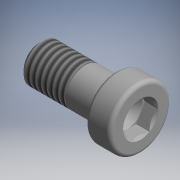
# Autodesk Inventor part: DIN-6912 - M10x20(F)
Saved by Autodesk Inventor 2017.3 (Build 213256000, 256)
## iProperties
Part Number: DIN-6912 - M10x20(F)
Material: Generic
Catalog Web Link: www.cadenas.de
Description: DIN-6912-Hexagon socket head cap screw with centre hole and low head
Vendor: FESTO
Document SubType Name: Modeling
Designer: partserver
Manufacturer: FESTO
Mass: 2.53132 g
Surface Area: 14.4572 cm^2
Volume: 2.53132 cm^3
Density: 1 g/cm^3
Appearance: PSOLRGB-192-192-192
Category: PARTsolutions
Company: FESTO
Title: DIN-6912 - M10x20(F)
Author: Cadenas PARTsolutions
Comments: Hexagon socket head cap screw with centre hole and low head
PSOL_IDENT_0: {$CADENAS_DATA\23d-libs\festo\zyl_zubeh\din_6912\din_6912.prj},183 {VTYP=3D},{NB=DIN-6912 - M10x20(F
PSOL_IDENT_1: )},{LINA=DIN-6912 - M10x20(F)},{NN=DIN-6912},{DATE=16.11.2017 11:29:57},{GEOMDATE=16.11.2017 11:29:4
PSOL_IDENT_2: 4},{VERSION=},{LINEID=430},{WBVAR=},{WBNUMERIC=}  {NB=DIN-6912 - M10x20(F)},{LINA=DIN-6912 - M10x20(
PSOL_IDENT_3: F)},{KT=L},{IDNR=},{NENN=M10x20},{D=10.000},{L=20.000},{DK=8.160},{LS=3.500},{LG=8.000},{DK1=16.000}
PSOL_IDENT_4: ,{DH=5.000},{K=6.500},{R=0.400},{V=1.000},{S=8.000},{T1=3.500},{T2=7.500},{F=1.020},{DA=11.200},{DW=
PSOL_IDENT_5: 15.030}
NB: DIN-6912 - M10x20(F)
NN: DIN-6912
NT: Hexagon socket head cap screw with centre hole and low head
NBSYN: DIN-6912 - $NENN.(F)
LINA: DIN-6912 - M10x20(F)
CATALOG: Festo
ROWDESC: M10x20
D: 10
L: 20
DK: 8.16
LS: 3.5
LG: 8
DK1: 16
DH: 5
K: 6.5
R: 0.4
V: 1
S: 8
T1: 3.5
T2: 7.5
F: 1.02
DA: 11.2
DW: 15.03
SUPPLIER: FESTO
ARTICLENO: DIN-6912 - M10x20(F)
BOMINFO: DIN-6912 - M10x20(F)
CREATOR: CADENAS GmbH
Autodesk Inventor part; units mm, degrees
sketch "Sketch_1" plane through (0, 0, 0) normal (0, 0, 1) x (1, 0, 0)
  line L0 (20, 0) -> (3.5, 0)
  line L1 (3.5, 0) -> (1, 2.5)
  line L2 (1, 2.5) -> (-1.5, 2.5)
  line L3 (-1.5, 2.5) -> (-3, 4)
  line L4 (-3, 4) -> (-5.8812, 4)
  line L5 (-5.8812, 4) -> (-6.5, 4.6188)
  line L6 (-6.5, 4.6188) -> (-6.5, 7)
  arc A0 (-5.5, 8) -> (-6.5, 7) centre (-5.5, 7) ccw
  line L7 (-5.5, 8) -> (-1, 8)
  arc A1 (0, 7) -> (-1, 8) centre (-1, 7) ccw
  line L8 (0, 7) -> (0, 5)
  line L9 (0, 5) -> (19.08, 5)
  line L10 (19.08, 5) -> (20, 4.08)
  line L11 (20, 4.08) -> (20, 0)
  line L12 (20, 0) -> (3.5, 0)
  constraints: 26 end point, 4 point on circle, 2 centre point
revolve "Revolution1" add sketch "Sketch_1" angle 360 about axis through (20, 0, 0) along (-1, 0, 0)
thread "Thread1" size "M10x1.5" class "6g" standard "ISO Metric profile" length 11.08
sketch "Sketch_2" plane through (-6.5, 0, 0) normal (1, 0, 0) x (0, 0, -1)
  line L0 (-4, -2.3094) -> (0, -4.6188)
  line L1 (0, -4.6188) -> (4, -2.3094)
  line L2 (4, -2.3094) -> (4, 2.3094)
  line L3 (4, 2.3094) -> (0, 4.6188)
  line L4 (0, 4.6188) -> (-4, 2.3094)
  line L5 (-4, 2.3094) -> (-4, -2.3094)
  constraints: 12 end point
extrude "Extrusion1" cut sketch "Sketch_2" along normal blind 3.5
ref_plane "MONTAGE_XY" through (0, 0, 0) normal (1, 0, 0) x (0, 0, -1)
ref_plane "MONTAGE_YZ" through (0, 0, 0) normal (0, 0, -1) x (0, 1, 0)
ref_plane "MONTAGE_ZX" through (0, 0, 0) normal (0, 1, 0) x (1, 0, 0)
ref_plane "Schrauben_punkt_XY" through (20, 0, 0) normal (-1, 0, 0) x (0, 0, -1)
ref_plane "Schrauben_punkt_YZ" through (20, 0, 0) normal (0, 0, -1) x (0, -1, 0)
ref_plane "Schrauben_punkt_ZX" through (20, 0, 0) normal (0, -1, 0) x (-1, 0, 0)
body "Solid1"
